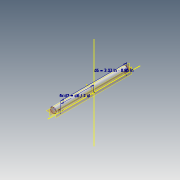
# Autodesk Inventor part: J005527
Saved by Autodesk Inventor 2015 SP1 (Build 190203100, 203)
## iProperties
Created: 2014-11-19
Material: ALUMINUM, 6061-T651
Vendor: HHMI: JRC - ID&F
Document SubType Name: Modeling
Designer: ARNOLDJ
Density: 2.7 g/cm^3
Description: NRB IDLER SHAFT
Project: COMMON
Mass: 9.72946 g
Surface Area: 10.4953 cm^2
Volume: 1.21618 cm^3
Appearance: Metal-AL-6061 (Machined)
Part Number: J005527
RuleStatus: InUse
AfterDocSave0: file://Part Number Cleaner
LAB/DEPT: COMMON
REQUESTING SCIENTIST: COMMON
SURFACE ROUGHNESS: N/A
DESIGN DEPARTMENT: HHMI: JRC - ID&F
SPECIAL FINISH: NONE
ALTERED ITEM PART NUMBER: 9061K32
ALTERED ITEM VENDOR: MCMASTER CARR
ALTERED ITEM DESCRIPTION: High-Strength 2024 Aluminum, Tight Tolerance, 3/16" Diameter
Author: ARNOLDJ
Revision Number: A
Autodesk Inventor part; units mm, degrees
ref_plane "Work Plane1" through (3.81, 0, 0) normal (1, 0, 0) x (0, 1, 0)
sketch "Sketch2" plane through (3.81, 0, 0) normal (1, 0, 0) x (0, 1, 0)
  line L0 (-38.5826, 0) -> (38.5826, 0) projected
  line L1 (0, 38.5826) -> (0, -38.5826) projected
  point P0 (0, 0)
  point P1 (0, 27.559)
  point P2 (0, -27.559)
  dimension "d6" = 55.118
  dimension "d7" = 27.559
  constraints: 1 midpoint
  measures "d6" distance of point (0, -27.559) point (0, 27.559)
  measures "d7" distance of point (0, 27.559) point (0, 0)
sketch "Sketch1" plane through (0, 0, 0) normal (0, 0, 1) x (1, 0, 0)
  circle A0 centre (0, 0) radius 2.3749
  dimension "d0" = 4.7498
  constraints: 1 centre point, 1 coincident
  measures "d0" diameter of A0
extrude "Extrusion1" add sketch "Sketch1" along normal mid plane 60.198
chamfer "Chamfer1" distance 0.254 angle 45 2 edges at (-2.3749, 0, 30.099) (-2.3749, 0, -30.099)
hole "Hole1" at (3.81, 0, 27.559) at (3.81, 0, -27.559) direction (-1, 0, 0) diameter 1.5748 end through all
equation "\"d7\" = 0.5 * d6"
body "Solid1"
